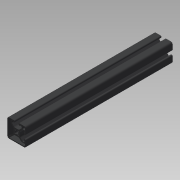
# Autodesk Inventor part: 1502-LS
Saved by Autodesk Inventor 2013 (Build 170138000, 138)
## iProperties
Company: 80/20 Inc.
Created: 2014-04-23
Part Number: 1502-LS
Material: Generic
Document SubType Name: Modeling
Density: 1 g/cm^3
Vendor: 80/20 Inc.
Engineer: Ross Bowman
Designer: Ross Bowman
Catalog Web Link: 8020.net
Material: 6105-T5 Aluminum
Author: Ross Bowman
Keywords: 80/20 , 8020 , T-Slot , Extrusion
Autodesk Inventor part; units mm, degrees
ref_plane "YZ Plane" through (0, 0, 0) normal (1, 0, 0) x (0, 1, 0)
ref_plane "XZ Plane" through (0, 0, 0) normal (0, 1, 0) x (-1, 0, 0)
ref_plane "XY Plane" through (0, 0, 0) normal (0, 0, 1) x (1, 0, 0)
sketch "Sketch1" plane through (0, 0, 0) normal (0, 0, 1) x (1, 0, 0)
  arc A0 (11.8618, 12.2428) -> (12.2428, 11.8618) centre (12.2428, 12.2428) ccw
  line L0 (11.8618, 16.8653) -> (11.8618, 12.2428)
  arc A1 (12.2428, 17.2463) -> (11.8618, 16.8653) centre (12.2428, 16.8653) ccw
  line L1 (14.4527, 17.2462) -> (12.2428, 17.2463)
  arc A2 (17.2466, 14.4522) -> (14.4527, 17.2462) centre (14.4526, 14.4522) ccw
  line L2 (17.2466, 12.2428) -> (17.2466, 14.4522)
  arc A3 (16.8656, 11.8618) -> (17.2466, 12.2428) centre (16.8656, 12.2428) ccw
  line L3 (12.2428, 11.8618) -> (16.8656, 11.8618)
  arc A4 (-6.8657, 2.742) -> (-8.2571, 6.1009) centre (-11.6155, 2.7421) ccw
  line L4 (-6.8659, -2.7433) -> (-6.8657, 2.742)
  arc A5 (-8.2569, -6.1016) -> (-6.8659, -2.7433) centre (-11.6157, -2.7432) ccw
  line L5 (-11.7735, -9.6186) -> (-8.2569, -6.1016)
  arc A6 (-11.7735, -9.6186) -> (-11.9967, -10.1574) centre (-11.2347, -10.1574) ccw
  line L6 (-11.9967, -10.4242) -> (-11.9967, -10.1574)
  arc A7 (-12.2199, -10.963) -> (-11.9967, -10.4242) centre (-12.7587, -10.4242) ccw
  line L7 (-16.5959, -15.3395) -> (-12.2199, -10.963)
  arc A8 (-17.2463, -15.0701) -> (-16.5959, -15.3395) centre (-16.8653, -15.0701) ccw
  line L8 (-17.2478, 14.452) -> (-17.2463, -15.0701)
  arc A9 (-14.4539, 17.2462) -> (-17.2478, 14.452) centre (-14.4538, 14.4522) ccw
  line L9 (-12.5802, 17.2463) -> (-14.4539, 17.2462)
  arc A10 (-12.1992, 16.8653) -> (-12.5802, 17.2463) centre (-12.5802, 16.8653) ccw
  line L10 (-12.1994, 11.3582) -> (-12.1992, 16.8653)
  arc A11 (-12.1994, 11.3582) -> (-11.2694, 9.1129) centre (-9.0244, 11.3581) ccw
  line L11 (-8.2571, 6.1009) -> (-11.2694, 9.1129)
  arc A12 (6.1009, -8.2571) -> (2.742, -6.8657) centre (2.7421, -11.6155) ccw
  line L12 (9.1129, -11.2694) -> (6.1009, -8.2571)
  arc A13 (9.1129, -11.2694) -> (11.3582, -12.1994) centre (11.3581, -9.0244) ccw
  line L13 (16.8653, -12.1992) -> (11.3582, -12.1994)
  arc A14 (17.2463, -12.5802) -> (16.8653, -12.1992) centre (16.8653, -12.5802) ccw
  line L14 (17.2462, -14.4539) -> (17.2463, -12.5802)
  arc A15 (14.452, -17.2478) -> (17.2462, -14.4539) centre (14.4522, -14.4538) ccw
  line L15 (-15.0701, -17.2463) -> (14.452, -17.2478)
  arc A16 (-15.3395, -16.5959) -> (-15.0701, -17.2463) centre (-15.0701, -16.8653) ccw
  line L16 (-10.963, -12.2199) -> (-15.3395, -16.5959)
  arc A17 (-10.4242, -11.9967) -> (-10.963, -12.2199) centre (-10.4242, -12.7587) ccw
  line L17 (-10.1574, -11.9967) -> (-10.4242, -11.9967)
  arc A18 (-10.1574, -11.9967) -> (-9.6186, -11.7735) centre (-10.1574, -11.2347) ccw
  line L18 (-6.1016, -8.2569) -> (-9.6186, -11.7735)
  arc A19 (-2.7433, -6.8659) -> (-6.1016, -8.2569) centre (-2.7432, -11.6157) ccw
  line L19 (2.742, -6.8657) -> (-2.7433, -6.8659)
  arc A20 (3.0179, -1.4014) -> (3.0178, 1.4017) centre (0, 0) ccw
  line L20 (4.3433, -2.7269) -> (3.0179, -1.4014)
  arc A21 (2.7269, -4.3433) -> (4.3433, -2.7269) centre (3.5351, -3.5351) ccw
  line L21 (1.4014, -3.0179) -> (2.7269, -4.3433)
  arc A22 (-1.4014, -3.0179) -> (1.4014, -3.0179) centre (0, 0) ccw
  line L22 (-2.7269, -4.3433) -> (-1.4014, -3.0179)
  arc A23 (-4.3433, -2.7269) -> (-2.7269, -4.3433) centre (-3.5351, -3.5351) ccw
  line L23 (-3.0179, -1.4014) -> (-4.3433, -2.7269)
  arc A24 (-3.0179, 1.4014) -> (-3.0179, -1.4014) centre (0, 0) ccw
  line L24 (-4.3433, 2.7269) -> (-3.0179, 1.4014)
  arc A25 (-2.7269, 4.3433) -> (-4.3433, 2.7269) centre (-3.5351, 3.5351) ccw
  line L25 (-1.4014, 3.0179) -> (-2.7269, 4.3433)
  arc A26 (1.4017, 3.0178) -> (-1.4014, 3.0179) centre (0, 0) ccw
  line L26 (2.6398, 4.2456) -> (1.4017, 3.0178)
  arc A27 (4.2456, 2.6398) -> (2.6398, 4.2456) centre (3.5351, 3.5351) ccw
  line L27 (3.0178, 1.4017) -> (4.2456, 2.6398)
  arc A28 (-6.858, 15.367) -> (-6.477, 14.986) centre (-6.477, 15.367) ccw
  line L28 (-6.477, 14.986) -> (-5.6388, 14.986)
  arc A29 (-5.6388, 14.986) -> (-4.064, 16.5608) centre (-5.6388, 16.5608) ccw
  line L29 (-4.064, 16.5608) -> (-4.064, 17.4752)
  arc A30 (-4.064, 17.4752) -> (-5.6388, 19.05) centre (-5.6388, 17.4752) ccw
  line L30 (-5.6388, 19.05) -> (-15.875, 19.05)
  arc A31 (-15.875, 19.05) -> (-19.05, 15.875) centre (-15.875, 15.875) ccw
  line L31 (-19.05, 15.875) -> (-19.05, -15.875)
  arc A32 (-19.05, -15.875) -> (-15.875, -19.05) centre (-15.875, -15.875) ccw
  line L32 (-15.875, -19.05) -> (15.875, -19.05)
  arc A33 (15.875, -19.05) -> (19.05, -15.875) centre (15.875, -15.875) ccw
  line L33 (19.05, -15.875) -> (19.05, -5.6388)
  arc A34 (19.05, -5.6388) -> (17.4752, -4.064) centre (17.4752, -5.6388) ccw
  line L34 (17.4752, -4.064) -> (16.5608, -4.064)
  arc A35 (16.5608, -4.064) -> (14.986, -5.6388) centre (16.5608, -5.6388) ccw
  line L35 (14.986, -5.6388) -> (14.986, -6.477)
  arc A36 (14.986, -6.477) -> (15.367, -6.858) centre (15.367, -6.477) ccw
  line L36 (15.367, -6.858) -> (15.4432, -6.858)
  arc A37 (15.8242, -7.239) -> (15.4432, -6.858) centre (15.4432, -7.239) ccw
  line L37 (15.8242, -7.239) -> (15.8242, -9.017)
  arc A38 (14.5542, -10.287) -> (15.8242, -9.017) centre (14.5542, -9.017) ccw
  line L38 (14.5542, -10.287) -> (12.9683, -10.287)
  arc A39 (12.0703, -9.915) -> (12.9683, -10.287) centre (12.9683, -9.017) ccw
  line L39 (12.0703, -9.915) -> (8.1222, -5.9669)
  arc A40 (6.731, -2.6083) -> (8.1222, -5.9669) centre (11.4808, -2.6083) ccw
  line L40 (6.731, -2.6083) -> (6.731, 2.6083)
  arc A41 (8.1222, 5.9669) -> (6.731, 2.6083) centre (11.4808, 2.6083) ccw
  line L41 (8.1222, 5.9669) -> (12.0703, 9.915)
  arc A42 (12.9683, 10.287) -> (12.0703, 9.915) centre (12.9683, 9.017) ccw
  line L42 (12.9683, 10.287) -> (14.5542, 10.287)
  arc A43 (15.8242, 9.017) -> (14.5542, 10.287) centre (14.5542, 9.017) ccw
  line L43 (15.8242, 9.017) -> (15.8242, 7.239)
  arc A44 (15.4432, 6.858) -> (15.8242, 7.239) centre (15.4432, 7.239) ccw
  line L44 (15.4432, 6.858) -> (15.367, 6.858)
  arc A45 (15.367, 6.858) -> (14.986, 6.477) centre (15.367, 6.477) ccw
  line L45 (14.986, 6.477) -> (14.986, 5.6388)
  arc A46 (14.986, 5.6388) -> (16.5608, 4.064) centre (16.5608, 5.6388) ccw
  line L46 (16.5608, 4.064) -> (17.4752, 4.064)
  arc A47 (17.4752, 4.064) -> (19.05, 5.6388) centre (17.4752, 5.6388) ccw
  line L47 (19.05, 5.6388) -> (19.05, 15.875)
  arc A48 (19.05, 15.875) -> (15.875, 19.05) centre (15.875, 15.875) ccw
  line L48 (15.875, 19.05) -> (5.6388, 19.05)
  arc A49 (5.6388, 19.05) -> (4.064, 17.4752) centre (5.6388, 17.4752) ccw
  line L49 (4.064, 17.4752) -> (4.064, 16.5608)
  arc A50 (4.064, 16.5608) -> (5.6388, 14.986) centre (5.6388, 16.5608) ccw
  line L50 (5.6388, 14.986) -> (6.477, 14.986)
  arc A51 (6.477, 14.986) -> (6.858, 15.367) centre (6.477, 15.367) ccw
  line L51 (6.858, 15.367) -> (6.858, 15.4432)
  arc A52 (7.239, 15.8242) -> (6.858, 15.4432) centre (7.239, 15.4432) ccw
  line L52 (7.239, 15.8242) -> (9.017, 15.8242)
  arc A53 (10.287, 14.5542) -> (9.017, 15.8242) centre (9.017, 14.5542) ccw
  line L53 (10.287, 14.5542) -> (10.287, 12.9683)
  arc A54 (9.915, 12.0703) -> (10.287, 12.9683) centre (9.017, 12.9683) ccw
  line L54 (9.915, 12.0703) -> (5.9669, 8.1222)
  arc A55 (2.6083, 6.731) -> (5.9669, 8.1222) centre (2.6083, 11.4808) ccw
  line L55 (2.6083, 6.731) -> (-2.6083, 6.731)
  arc A56 (-5.9669, 8.1222) -> (-2.6083, 6.731) centre (-2.6083, 11.4808) ccw
  line L56 (-5.9669, 8.1222) -> (-9.915, 12.0703)
  arc A57 (-10.287, 12.9683) -> (-9.915, 12.0703) centre (-9.017, 12.9683) ccw
  line L57 (-10.287, 12.9683) -> (-10.287, 14.5542)
  arc A58 (-9.017, 15.8242) -> (-10.287, 14.5542) centre (-9.017, 14.5542) ccw
  line L58 (-9.017, 15.8242) -> (-7.239, 15.8242)
  arc A59 (-6.858, 15.4432) -> (-7.239, 15.8242) centre (-7.239, 15.4432) ccw
  line L59 (-6.858, 15.4432) -> (-6.858, 15.367)
  constraints: 120 end point, 120 point on circle, 60 centre point
extrude "Extrusion1" add sketch "Sketch1" against normal blind 304.8
body "Solid1"
